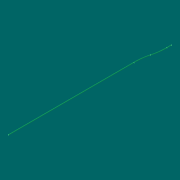
# Autodesk Inventor part: Fiber Loop
Saved by Autodesk Inventor 2016 SP2 (Build 200236200, 236)
## iProperties
Created: 2015-08-17
Part Number: Fiber Loop
Material: Glass
Document SubType Name: Modeling
Designer: Cosmic
Density: 2.18 g/cm^3
Appearance: Clear - Green 1
Author: Cosmic
Autodesk Inventor part; units mm, degrees
note: some values were not read from the file. Left out: dimensions or parameters whose unit could not be read.
ref_plane "YZ Plane" through (0, 0, 0) normal (1, 0, 0) x (0, 1, 0)
ref_plane "XZ Plane" through (0, 0, 0) normal (0, 1, 0) x (-1, 0, 0)
ref_plane "XY Plane" through (0, 0, 0) normal (0, 0, 1) x (1, 0, 0)
sketch "Sketch3" plane through (0, 0, 0) normal (1, 0, 0) x (0, 1, 0)
  line L0 (0, 0) -> (151.2449, 0)
  arc A0 (171.087, -2.2145) -> (151.2449, 0) centre (151.2449, -90) ccw
  arc A1 (171.087, -2.2145) -> (190.929, -4.429) centre (190.929, 85.571) ccw
  line L1 (190.929, -4.429) -> (196.5, -4.429)
  line L2 (0, 1) -> (151.2449, 1)
  arc A2 (171.3074, -1.2391) -> (151.2449, 1) centre (151.2449, -90) ccw
  arc A3 (171.3074, -1.2391) -> (190.929, -3.429) centre (190.929, 85.571) ccw
  line L3 (190.929, -3.429) -> (196.5, -3.429)
  line L4 (196.5, -4.429) -> (196.5, -3.429)
  line L5 (0, 0) -> (0, 1)
  dimension "d42" = 90
  dimension "d43" = 90
  dimension "d44" = 4.429
  dimension "d45" = 5.571
  dimension "d46" = 1
  dimension "d50" = 196.5
  constraints: 12 end point, 8 point on circle, 4 centre point, 3 tangent, 2 horizontal, 1 coincident, 1 parallel, 1 vertical, 3 other
  measures "d42" radius of A0
  measures "d43" radius of A1
  measures "d44" distance between parallel lines of L0 L1
  measures "d45" distance of L1.start L1.end
  measures "d46" distance between parallel lines of L1 L3
  measures "d50" distance between parallel lines of L5 L4
extrude "fiberBase" add sketch "Sketch3" along normal blind 1
fillet "round" radius 0.5 16 edges at (1, 181.0573, -2.8798) (1, 161.3385, 0.4385) (1, 75.6225, 1) (1, 193.7145, -3.429) (0, 181.0573, -2.8798) (0, 161.3385, 0.4385) (0, 75.6225, 1) (0, 193.7145, -3.429) (0, 180.9464, -3.8737) (0, 161.2276, -0.5553) (0, 75.6225, 0) (0, 193.7145, -4.429) (1, 180.9464, -3.8737) (1, 161.2276, -0.5553) (1, 75.6225, 0) (1, 193.7145, -4.429)
equation "\"d42\" = curvatureRadius"
equation "\"d43\" = curvatureRadius"
equation "\"d44\" = deepTrackDepth - shallowTrackDepth"
equation "\"d45\" = deepTrackDepth"
equation "\"d46\" = opticalFiberDiameter"
equation "\"d50\" = -scintillatorEdgeClearence + scintillatorHeight - 0.5 * opticalFiberDiameter"
equation "\"d47\" = opticalFiberDiameter"
equation "\"d49\" = 0.5 * opticalFiberDiameter"
equation "\"OpticalFiberDiameter\" = 1"
equation "\"OpticalFiberClearence\" = 0.071"
equation "\"ScintillatorEdgeClearence\" = 3"
equation "\"MPPCDepth\" = 1"
equation "\"LoopLargeTrackRatio\" = 1.1"
equation "\"d24\" = 0.05"
equation "\"d25\" = 1"
equation "\"d32\" = 0.05"
equation "\"d33\" = 1"
equation "\"FiberSensorClerence\" = 0.5"
equation "\"SmallTrackDiameter\" = 175"
equation "\"ShallowTrackDepth\" = 1.142"
equation "\"MPPCClearence\" = 0.075"
equation "\"MPPCSensorClearence\" = 1.45"
equation "\"MPPCSensorOffsett\" = 2.105"
equation "\"MPPCWidth\" = 5.9"
equation "\"MPPCHeight\" = 6.55"
equation "\"FiberEdgeOffsett\" = 5"
equation "\"LongFiberAngle\" = 30deg"
equation "\"ShortFiberAngle\" = 78deg"
equation "\"MountingScrewOffsett\" = 9"
equation "\"MountingScrewDepth\" = 4"
equation "\"DeepTrackDepth\" = 5.571"
equation "\"FoilThickness\" = 0.2"
equation "\"silveringThickness\" = 0.2"
equation "\"mppcMountDepth\" = 6.35"
equation "\"curvatureRadius\" = 90"
equation "\"shallowTrackDepth\" = 1.142"
equation "\"deepTrackDepth\" = 5.571"
equation "\"fiberEdgeOffsett\" = 5"
equation "\"scintillatorEdgeClearence\" = 3"
equation "\"opticalFiberDiameter\" = 1"
equation "\"opticalFiberClearence\" = 0.071"
equation "\"scintillatorHeight\" = 200"
body "Solid2"
